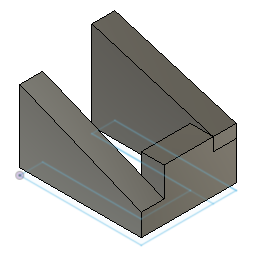
gum holder (Autodesk Fusion 360 design; units mm, degrees)
Autodesk Fusion 360 part; units mm, degrees
sketch "Sketch1" plane through (0, 0, 0) normal (0, 0, 1) x (1, 0, 0)
  line L0 (0, 0) -> (0, 7)
  line L1 (37, 29) -> (0, 29)
  line L2 (0, 29) -> (0, 22)
  line L3 (0, 22) -> (30, 22)
  line L4 (30, 22) -> (30, 7)
  line L5 (0, 7) -> (30, 7)
  line L6 (37, 0.0498) -> (37, 29)
  line L7 (0, 7) -> (30, 7)
  line L8 (30, 22) -> (0, 22)
  line L9 (0, 29) -> (37, 29)
  line L10 (0, 0) -> (37, 0.0498)
  line L11 (30, 22) -> (37.000001, 22)
  dimension "d2" = 7
  dimension "d12" = 15
  dimension "d13" = 7
  dimension "d14" = 30
  dimension "d15" = 7
  constraint coincident L0.start L10.start
  constraint perpendicular L1 L2
  constraint perpendicular L2 L3
  constraint perpendicular L4 L5
  constraint perpendicular L6 L11
  measures "d2" distance of L0.start L0.end
  measures "d12" distance of L5 L8
  measures "d13" distance of L1.end L2.end
  measures "d14" distance of L0.end L4.end
  measures "d15" distance of L4 L6
extrude "Extrude1" add sketch "Sketch1" along normal blind 8 contours L0 L4 L5 L6 L7 L10 L11 | L1 L2 L3 L6 L8 L9 L11 picked at (22.333333, 2.349933) picked at (22.333333, 26.666667)
ref_plane "WorkPlane1" through (0, 0, 0) normal (0, 1, 0) x (0, 0, 1)
sketch "Sketch2" plane through (0, 0, 0) normal (0, 1, 0) x (1, 0, 0)
extrude "Extrude2" cut 1 faces at (22.333333, 26.666667, 8) along direction (0, 0, -1) blind 8
extrude "Extrude3" add sketch "Sketch1" along normal blind 29 contours L0 L4 L5 L6 L7 L10 L11 | L1 L2 L3 L6 L8 L9 L11 picked at (22.333333, 2.349933) picked at (22.333333, 26.666667)
extrude "Extrude4" cut 1 faces at (22.333333, 26.666667, 29) along direction (0, 0, -1) blind 29
extrude "Extrude5" add sketch "Sketch1" along normal blind 29 contours L1 L2 L3 L6 L8 L9 L11 picked at (22.333333, 26.666667)
extrude "Extrude6" add sketch "Sketch1" along normal blind 24 contours L0 L4 L5 L6 L7 L10 L11 picked at (22.333333, 2.349933)
ref_plane "WorkPlane2" through (18.5, 29, 14.5) normal (0, 1, 0) x (-1, 0, 0)
sketch "Sketch3" plane through (18.5, 29, 14.5) normal (0, 1, 0) x (1, 0, 0)
  line L0 (-18.5, 14.5) -> (18.5, 14.5)
  line L1 (-18.5, -14.5) -> (18.4993, 0.781198)
  line L2 (18.5, 14.5) -> (-18.5, 14.5)
  line L3 (-18.5, -14.5) -> (18.502182, -14.499999)
  line L4 (18.502182, -14.499999) -> (18.4993, 0.781198)
  dimension "d24" = 22.44127
  measures "d24" angle of L1 L2
extrude "Extrude7" cut sketch "Sketch3" against normal blind 7 contours L1 L3 L4 picked at (6.167161, -9.406267)
extrude "Extrude8" cut 1 faces at (36.999533, 26.666667, 14.956744) along direction (0.99999998, 0, -0.00018863) blind 1
sketch "Sketch4" plane through (0, 0, 0) normal (0, 1, 0) x (1, 0, 0)
  line L0 (0, 0) -> (37, 0)
  line L1 (37.000002, -8.74) -> (0, -24.000001)
  line L2 (37.000001, -24) -> (37.000002, -8.74)
  line L3 (0, -24.000001) -> (37.000001, -24)
extrude "Extrude9" cut sketch "Sketch4" along normal blind 7 contours L1 L2 L3 picked at (24.666667, -18.913334)
extrude "Extrude10" cut 1 faces at (34.666667, 12, 24) along direction (0, 0, -1) blind 10.28
extrude "Extrude11" add 2 faces at (36.998567, 22, 13.719601) (34.665467, 12, 13.72) along direction (0, 0, 1) blind 4
ref_plane "WorkPlane3" through (0, 0, 0) normal (0, 1, 0) x (0, 0, 1)
sketch "Sketch5" plane through (0, 0, 0) normal (0, 1, 0) x (1, 0, 0)
sketch "Sketch6" plane through (0, 29, 0) normal (0, 1, 0) x (-1, 0, 0)
  line L0 (-36.9993, 13.718802) -> (-37, 13.718802)
  line L1 (-37, 13.718802) -> (-37, 0)
  line L2 (-37, 0) -> (0, 0)
  line L3 (0, 0) -> (0, 29)
  line L4 (0, 29) -> (-36.9993, 13.718802)
  line L5 (-36.9993, 13.718802) -> (-37.000055, 17.720968)
  line L6 (-37.000055, 17.720968) -> (0, 29)
  line L7 (0, 29) -> (-36.9993, 13.718802)
  constraint perpendicular L0 L5
  constraint coincident L3.end L4.start
extrude "Extrude12" add sketch "Sketch6" against normal blind 7 contours L4 L5 L6 L7 picked at (-24.666451, 20.14659)
extrude "Extrude13" cut sketch "Sketch1" along normal blind 2 contours L1 L2 L3 L6 L8 L9 L11 picked at (22.333333, 26.666667)
extrude "Extrude14" cut sketch "Sketch1" along normal blind 2 contours L0 L4 L5 L6 L7 L10 L11 picked at (22.333333, 2.349933)
